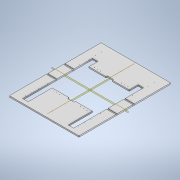
# Autodesk Inventor part: top_part
Saved by Autodesk Inventor 2020 (Build 240168000, 168)
## iProperties
Created: 2019-12-27
Part Number: top_part
Material: Générique
Document SubType Name: Modeling
Designer: damien
Density: 1 g/cm^3
Appearance: Par défaut
Author: damien
Autodesk Inventor part; units mm, degrees
ref_plane "YZ Plane" through (0, 0, 0) normal (1, 0, 0) x (0, 1, 0)
ref_plane "XZ Plane" through (0, 0, 0) normal (0, 1, 0) x (-1, 0, 0)
ref_plane "XY Plane" through (0, 0, 0) normal (0, 0, 1) x (1, 0, 0)
sketch "Esquisse1" plane through (0, 0, 0) normal (0, 1, 0) x (-1, 0, 0)
  line L0 (-550, -725) -> (550, -725)
  line L1 (550, -725) -> (550, 725)
  line L2 (550, 725) -> (-550, 725)
  line L3 (-550, 725) -> (-550, -725)
  line L4 (-550, -725) -> (550, 725) construction
  line L5 (550, -725) -> (-550, 725) construction
  point P0 (0, 0)
  dimension "d0" = 1450
  dimension "d1" = 1100
  constraints: 12 end point, 2 midpoint, 2 parallel, 1 horizontal, 1 perpendicular
  measures "d0" distance of L0.end L1.end
  measures "d1" distance of L1.end L2.end
extrude "Extrusion1" add sketch "Esquisse1" along normal blind 21
sketch "Esquisse2" plane through (0, 21, 0) normal (0, 1, 0) x (1, 0, 0)
  line L0 (-404, -662) -> (-404, 444)
  line L1 (-404, 444) -> (-318, 444)
  line L2 (-318, 444) -> (-318, 302)
  line L3 (-318, 302) -> (318, 302)
  line L4 (318, 302) -> (318, 444)
  line L5 (318, 444) -> (404, 444)
  line L6 (404, 444) -> (404, -662)
  line L7 (404, -662) -> (318, -662)
  line L8 (318, -662) -> (318, -281)
  line L9 (318, -281) -> (-318, -281)
  line L10 (-318, -281) -> (-318, -662)
  line L11 (-318, -662) -> (-404, -662)
  line L12 (550, -725) -> (550, 725) projected
  line L13 (-550, 725) -> (-550, -725) projected
  line L14 (-550, -725) -> (550, -725) projected
  line L15 (550, 725) -> (-550, 725) projected
  line L16 (-550, 0) -> (-404, 0) construction
  line L17 (550, 0) -> (404, 0) construction
  point P0 (0, 0)
  dimension "d4" = 1106
  dimension "d5" = 86
  dimension "d7" = 583
  dimension "d8" = 142
  dimension "d55" = 636
  dimension "d56" = 281
  constraints: 28 end point, 9 point on line, 8 perpendicular, 3 equal length, 2 midpoint, 2 vertical
  measures "d4" distance of L5.end L6.end
  measures "d5" distance of L6.end L7.end
  measures "d7" distance between parallel lines of L3 L9
  measures "d8" distance of L3.end L4.end
  measures "d55" distance between parallel lines of L8 L10
  measures "d56" distance between parallel lines of L15 L1
extrude "Extrusion2" cut sketch "Esquisse2" against normal blind 21.1 contours L0 L1 L2 L3 L4 L5 L6 L7 L8 L9 L10 L11
sketch "Esquisse3" plane through (-550, 0, 575) normal (1, 0, 0) x (0, 0, -1)
  line L0 (-87, 21) -> (1019, 21) projected
  line L1 (432, 21) -> (456, 21)
  line L2 (456, 21) -> (456, 11)
  line L3 (456, 11) -> (432, 11)
  line L4 (432, 11) -> (432, 21)
  line L5 (-150, 0) -> (-150, 21) projected
  line L6 (703, 21) -> (727, 21)
  line L7 (727, 21) -> (727, 11)
  line L8 (727, 11) -> (703, 11)
  line L9 (703, 11) -> (703, 21)
  line L10 (877, 21) -> (877, 0) projected
  line L11 (294, 21) -> (294, 0) projected
  point P0 (575, 0)
  point P1 (456, 21)
  dimension "d14" = 24
  dimension "d15" = 10
  dimension "d17" = 24
  dimension "d57" = 150
  dimension "d58" = 138
  constraints: 16 end point, 4 parallel, 2 horizontal, 2 perpendicular, 2 point on line, 1 collinear
  measures "d14" distance of L2.end L3.end
  measures "d15" distance of L1.end L2.end
  measures "d17" distance of L7.end L8.end
  measures "d57" distance between parallel lines of L10 L7
  measures "d58" distance between parallel lines of L11 L4
extrude "Extrusion3" cut sketch "Esquisse3" along normal blind 1500
sketch "Esquisse4" plane through (0, 21, 0) normal (0, 1, 0) x (1, 0, 0)
  line L0 (318, 302) -> (-318, 302) projected
  line L1 (-50, 302) -> (50, 302)
  line L2 (50, 302) -> (50, 322)
  line L3 (50, 322) -> (-50, 322)
  line L4 (-50, 322) -> (-50, 302)
  line L5 (-318, -281) -> (318, -281) projected
  line L6 (-50, -281) -> (50, -281)
  line L7 (50, -281) -> (50, -304)
  line L8 (50, -304) -> (-50, -304)
  line L9 (-50, -304) -> (-50, -281)
  line L10 (-318, 444) -> (-318, 302) projected
  line L11 (318, 302) -> (318, 444) projected
  point P0 (0, 0)
  point P1 (50, 302)
  point P2 (0, 302)
  dimension "d20" = 23
  dimension "d21" = 100
  dimension "d50" = 20
  constraints: 16 end point, 4 parallel, 4 point on line, 2 horizontal, 2 midpoint, 2 perpendicular
  measures "d20" distance of L6.end L7.end
  measures "d21" distance of L2.end L3.end
  measures "d50" distance of L1.end L2.end
extrude "Extrusion4" cut sketch "Esquisse4" against normal blind 100
fillet "Congé1" radius 2 8 edges at (50, 10.5, -322) (50, 10.5, -302) (-50, 10.5, -322) (-50, 10.5, -302) (-50, 10.5, 281) (-50, 10.5, 304) (50, 10.5, 304) (50, 10.5, 281)
sketch "Esquisse5" plane through (0, 21, 0) normal (0, 1, 0) x (1, 0, 0)
  circle A0 centre (0, 502) radius 2.25
  circle A1 centre (0, 402) radius 2.25
  line L0 (-550, 725) -> (-550, -725) projected
  line L1 (550, -725) -> (550, 725) projected
  circle A2 centre (0, 602) radius 2.25
  line L2 (-318, 302) -> (-52, 302) projected
  circle A3 centre (417, 602) radius 2.25
  circle A4 centre (417, 502) radius 2.25
  circle A5 centre (417, 402) radius 2.25
  circle A6 centre (-417, 402) radius 2.25
  circle A7 centre (-417, 502) radius 2.25
  circle A8 centre (-417, 602) radius 2.25
  circle A9 centre (-417, 252) radius 2.25
  circle A10 centre (417, 252) radius 2.25
  line L3 (0, 402) -> (0, 322) construction
  line L4 (48, 322) -> (-48, 322) projected
  point P0 (0, 0)
  point P1 (-550, 152)
  dimension "d29" = 100
  dimension "d30" = 100
  dimension "d32" = 100
  dimension "d35" = 133
  dimension "d36" = 133
  dimension "d51" = 150
  dimension "d52" = 4.5
  constraints: 11 centre point, 11 equal radius, 8 vertical alignment, 7 horizontal alignment, 2 end point, 1 midpoint, 1 vertical
  measures "d29" distance of A0.centre L3.start
  measures "d30" distance of A0.centre A2.centre
  measures "d32" distance from line of L3.start L2
  measures "d35" distance from line of L1 A4.centre
  measures "d36" distance from line of L0 A6.centre
  measures "d51" distance of A9.centre A6.centre
  measures "d52" diameter of A1
extrude "Extrusion5" cut sketch "Esquisse5" against normal blind 100
mirror "Symétrie1" about plane through (0, 0, 0) normal (0, 0, 1) of "Extrusion5"
sketch "Esquisse6" plane through (0, 21, 0) normal (0, 1, 0) x (1, 0, 0)
  circle A0 centre (-265.5, -313) radius 2.25
  line L0 (-318, -662) -> (-318, -281) projected
  line L1 (-318, -313) -> (318, -313) construction
  line L2 (318, -662) -> (318, -281) projected
  line L3 (48, -304) -> (-48, -304) projected
  circle A1 centre (-215.5, -313) radius 2.25
  circle A2 centre (-165.5, -313) radius 2.25
  line L4 (-48, -304) -> (48, -304) projected
  line L5 (0, -304) -> (0, -725) construction
  line L6 (-550, -725) -> (550, -725) projected
  circle A3 centre (265.5, -313) radius 2.25
  circle A4 centre (215.5, -313) radius 2.25
  circle A5 centre (165.5, -313) radius 2.25
  point P0 (0, 0)
  dimension "d37" = 4.5
  dimension "d38" = 9
  dimension "d39" = 52.5
  dimension "d42" = 50
  constraints: 6 centre point, 4 end point, 3 midpoint, 3 point on line, 3 symmetric about line, 2 horizontal, 1 vertical, 7 other
  measures "d37" diameter of A0
  measures "d38" distance between parallel lines of L1 L3
  measures "d39" distance from line of L0 A0.centre
  measures "d42" distance of A0.centre A1.centre
extrude "Extrusion6" cut sketch "Esquisse6" against normal blind 100
sketch "Esquisse7" plane through (0, 21, 0) normal (0, 1, 0) x (1, 0, 0)
  circle A0 centre (265.5, 334) radius 2.25
  circle A1 centre (215.5, 334) radius 2.25
  circle A2 centre (165.5, 334) radius 2.25
  circle A3 centre (-165.5, 334) radius 2.25
  circle A4 centre (-215.5, 334) radius 2.25
  circle A5 centre (-265.5, 334) radius 2.25
  line L0 (318, 302) -> (318, 444) projected
  circle A6 centre (265.5, -313) radius 2.25 projected
  line L1 (50, 320) -> (50, 304) projected
  circle A7 centre (-265.5, -313) radius 2.25 projected
  line L2 (-52, -281) -> (-318, -281) projected
  line L3 (-318, 302) -> (-52, 302) projected
  point P0 (0, 0)
  dimension "d60" = 50
  dimension "d61" = 50
  dimension "d62" = 115.5
  dimension "d63" = 50
  dimension "d64" = 50
  dimension "d66" = 32
  constraints: 6 centre point, 6 equal radius, 5 horizontal alignment, 2 vertical alignment
  measures "d60" distance of A0.centre A1.centre
  measures "d61" distance of A1.centre A2.centre
  measures "d62" distance from line of A2.centre L1
  measures "d63" distance of A4.centre A5.centre
  measures "d64" distance of A3.centre A4.centre
  measures "d66" distance from line of L3 A5.centre
fillet "Congé2" radius 5 4 edges at (550, 10.5, -725) (-550, 10.5, -725) (-550, 10.5, 725) (550, 10.5, 725)
ref_plane "Plan de construction2" through (0, 21, -128) normal (-1, 0, 0) x (0, 0, 1)
extrude "Extrusion7" cut sketch "Esquisse7" against normal blind 21 contours A0 | A1 | A2 | A3 | A4 | A5
ref_plane "Plan de construction1" through (0, 0, 0) normal (0, 0, 1) x (1, 0, 0)
